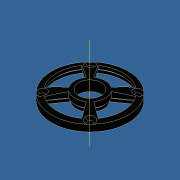
# Autodesk Inventor part: encoder_kappe_s
Saved by Autodesk Inventor 2016 (Build 200138000, 138)
## iProperties
Created: 2016-04-07
Part Number: encoder_kappe_s
Material: ABS-Kunststoff
Document SubType Name: Modeling
Designer: 4ndreas
Density: 1.06 g/cm^3
Appearance: Glatt - schwarz
Mass: 4.39722 g
Surface Area: 43.6627 cm^2
Volume: 4.14832 cm^3
Author: 4ndreas
Autodesk Inventor part; units mm, degrees
ref_plane "YZ Plane" through (0, 0, 0) normal (1, 0, 0) x (0, 1, 0)
ref_plane "XZ Plane" through (0, 0, 0) normal (0, 1, 0) x (-1, 0, 0)
ref_plane "XY Plane" through (0, 0, 0) normal (0, 0, 1) x (1, 0, 0)
sketch "Skizze1" plane through (0, 0, 0) normal (0, 0, 1) x (1, 0, 0)
  circle A0 centre (0, 0) radius 25.325
  circle A1 centre (0, 0) radius 7.5
  arc A2 (-8.291803, 5.766803) -> (-8.291803, -5.766803) centre (0, 0) ccw
  arc A3 (-17.917682, 12.461432) -> (-17.917682, -12.461432) centre (0, 0) ccw
  circle A4 centre (-16, 16) radius 1.6
  line L0 (-16, 16) -> (0, 16) construction
  line L1 (0, 16) -> (0, 0) construction
  line L2 (0, 0) -> (-16, 0) construction
  line L3 (-16, 0) -> (-16, 16) construction
  line L4 (-17.917682, 12.461432) -> (-8.291803, 5.766803)
  line L5 (-17.917682, -12.461432) -> (-8.291803, -5.766803)
  circle A5 centre (-16, 16) radius 4 construction
  line L6 (-16, 16) -> (0, 0) construction
  line L7 (0, 0) -> (-20.791079, 14.459829) construction
  line L8 (-12.461432, -17.917682) -> (-5.766803, -8.291803)
  circle A6 centre (-16, -16) radius 1.6
  arc A7 (-12.461432, -17.917682) -> (12.461432, -17.917682) centre (0, 0) ccw
  arc A8 (-5.766803, -8.291803) -> (5.766803, -8.291803) centre (0, 0) ccw
  line L9 (12.461432, -17.917682) -> (5.766803, -8.291803)
  line L10 (17.917682, -12.461432) -> (8.291803, -5.766803)
  circle A9 centre (16, -16) radius 1.6
  arc A10 (17.917682, -12.461432) -> (17.917682, 12.461432) centre (0, 0) ccw
  arc A11 (8.291803, -5.766803) -> (8.291803, 5.766803) centre (0, 0) ccw
  line L11 (17.917682, 12.461432) -> (8.291803, 5.766803)
  line L12 (12.461432, 17.917682) -> (5.766803, 8.291803)
  circle A12 centre (16, 16) radius 1.6
  arc A13 (12.461432, 17.917682) -> (-12.461432, 17.917682) centre (0, 0) ccw
  arc A14 (5.766803, 8.291803) -> (-5.766803, 8.291803) centre (0, 0) ccw
  line L13 (-12.461432, 17.917682) -> (-5.766803, 8.291803)
  dimension "d2" = 50.65
  dimension "d3" = 32
  dimension "d4" = 3.2
  dimension "d5" = 15
  dimension "d6" = 2.6
  dimension "d7" = 3.5
  dimension "d8" = 360
  dimension "d9" = 8
  constraints: 28 end point, 16 point on circle, 14 centre point, 9 coincident, 2 parallel, 2 perpendicular, 2 tangent, 1 horizontal, 1 point on line, 53 other
  measures "d3" diameter of L3 L1
  measures "d4" diameter of A4
  measures "d5" diameter of A1
  measures "d6" radial gap between concentric circles of A1 A2
  measures "d9" diameter of A5
extrude "Extrusion1" add sketch "Skizze1" along normal blind 5
ref_plane "Arbeitsebene1" through (-16, 16, 0) normal (0.7071068, 0.7071068, 0) x (0, 0, 1)
sketch "Skizze2" plane through (-16, 16, 0) normal (0.7071068, 0.7071068, 0) x (0, 0, 1)
  line L0 (5, 1.6) -> (0, 1.6)
  line L1 (0, 1.6) -> (0, 15.127417)
  line L2 (0, 15.127417) -> (5, 15.127417)
  line L3 (5, 15.127417) -> (5, 1.6)
  line L4 (0, 43.654834) -> (5, 43.654834)
  line L5 (5, 43.654834) -> (5, 30.127417)
  line L6 (5, 30.127417) -> (0, 30.127417)
  line L7 (0, 30.127417) -> (0, 43.654834)
  line L8 (0, 47.952417) -> (5, 47.952417)
  line L9 (5, 47.952417) -> (5, 46.854834)
  line L10 (5, 46.854834) -> (0, 46.854834)
  line L11 (0, 46.854834) -> (0, 47.952417)
  line L12 (5, -2.697583) -> (0, -2.697583)
  line L13 (0, -2.697583) -> (0, -1.6)
  line L14 (0, -1.6) -> (5, -1.6)
  line L15 (5, -1.6) -> (5, -2.697583)
  line L16 (-150.550047, 22.627417) -> (31.652407, 22.627417)
  arc A0 (5, 22.627417) -> (2.5, 47.952417) centre (-124.521125, 22.627417) ccw
  line L17 (5, 30.127417) -> (5, 15.127417)
  line L18 (2.5, 47.952417) -> (5, 47.952417)
  line L19 (5, 47.952417) -> (5, 22.627417)
  point P0 (0, 22.627417)
  dimension "d12" = 2.5
  constraints: 4 end point, 2 midpoint, 2 point on circle, 2 tangent, 1 centre point, 1 horizontal, 1 perpendicular, 1 point on line
  measures "d12" distance from line of L18.start L9
revolve "Umdrehung1" cut sketch "Skizze2" angle 360 about axis through (0, 0, 0) along (0, 0, 1) contours A0 L10 L19 L4 | L4 L5 L6 A0 | L6 L17 A0 | A0 L8 L9 L10
chamfer "Fase1" distance 1 angle 45 16 edges at (-21.825, 0, 0) (-13.1047, -9.1141, 0) (0, -21.825, 0) (-9.1141, -13.1047, 0) (9.1141, -13.1047, 0) (13.1047, -9.1141, 0) (21.825, 0, 0) (13.1047, 9.1141, 0) (0, 21.825, 0) (9.1141, 13.1047, 0) (-9.1141, 13.1047, 0) (-13.1047, 9.1141, 0) (-10.1, 0, 0) (0, -10.1, 0) (10.1, 0, 0) (0, 10.1, 0)
chamfer "Fase2" distance 1.5 angle 45 6 edges at (17.4789, -16.6106, 2.7357) (14.8686, -17.1314, 2.9981) (16.6218, -14.5258, 3.105) (-17.6, -15.9999, 2.7972) (-17.6, 15.9999, 2.7972) (14.4, 15.9999, 3.1987)
sketch "Skizze3" plane through (0, 0, 0) normal (0, 0, -1) x (-1, 0, 0)
  line L0 (-6.854616, 5.985335) -> (-18.149689, 13.84086)
  arc A0 (-6.854616, 5.985335) -> (-6.854616, -5.985335) centre (0, 0) ccw
  line L1 (-18.149689, -13.84086) -> (-6.854616, -5.985335)
  arc A1 (-18.149689, 13.84086) -> (-18.149689, -13.84086) centre (0, 0) ccw
  line L2 (6.854616, -5.985335) -> (18.149689, -13.84086)
  arc A2 (6.854616, -5.985335) -> (6.854616, 5.985335) centre (0, 0) ccw
  line L3 (18.149689, 13.84086) -> (6.854616, 5.985335)
  arc A3 (18.149689, -13.84086) -> (18.149689, 13.84086) centre (0, 0) ccw
  circle A4 centre (0, 0) radius 7.5
  circle A5 centre (-16, 16) radius 1.6
  circle A6 centre (16, -16) radius 1.6
  circle A7 centre (16, 16) radius 1.6
  circle A8 centre (-16, -16) radius 1.6
  circle A9 centre (0, 0) radius 25.325
  line L4 (-5.985335, -6.854616) -> (-13.84086, -18.149689)
  arc A10 (-5.985335, -6.854616) -> (5.985335, -6.854616) centre (0, 0) ccw
  line L5 (13.84086, -18.149689) -> (5.985335, -6.854616)
  arc A11 (-13.84086, -18.149689) -> (13.84086, -18.149689) centre (0, 0) ccw
  line L6 (5.985335, 6.854616) -> (13.84086, 18.149689)
  arc A12 (5.985335, 6.854616) -> (-5.985335, 6.854616) centre (0, 0) ccw
  line L7 (-13.84086, 18.149689) -> (-5.985335, 6.854616)
  arc A13 (13.84086, 18.149689) -> (-13.84086, 18.149689) centre (0, 0) ccw
extrude "Extrusion2" add sketch "Skizze3" along normal blind 2
